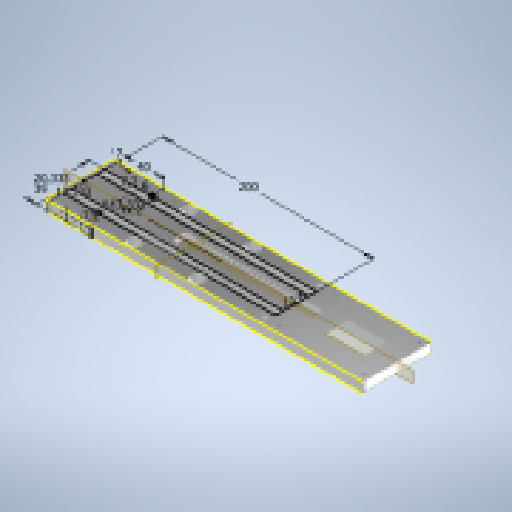
# Autodesk Inventor part: SchlittenS
Saved by Autodesk Inventor 2025 (Build 290162010, 162A)
## iProperties
Created: 2024-11-19
Part Number: SchlittenS
Material: Aluminium 6061(1)
Document SubType Name: Modeling
Designer: Admin
Density: 2.7 g/cm^3
Appearance: Aluminium - flach(1)
Author: Admin
Autodesk Inventor part; units mm, degrees
ref_plane "YZ Plane" through (0, 0, 0) normal (1, 0, 0) x (0, 1, 0)
ref_plane "XZ Plane" through (0, 0, 0) normal (0, 1, 0) x (-1, 0, 0)
ref_plane "XY Plane" through (0, 0, 0) normal (0, 0, 1) x (1, 0, 0)
sketch "Skizze1" plane through (0, 0, 0) normal (0, 0, 1) x (1, 0, 0)
  line L0 (300, 65) -> (0, 65)
  line L1 (0, 65) -> (0, 0)
  line L2 (0, 0) -> (300, 0)
  line L3 (300, 0) -> (300, 65)
  line L4 (144, -16) -> (70, -16)
  line L5 (70, -16) -> (70, 81)
  line L6 (70, 81) -> (144, 81)
  line L7 (144, 81) -> (144, -16)
  dimension "d0" = 300
  dimension "d1" = 65
  dimension "d220" = 74
  dimension "d221" = 16
  dimension "d222" = 16
  dimension "d223" = 70
  constraints: 16 end point, 4 parallel, 2 perpendicular, 1 horizontal, 1 vertical, 1 other
  measures "d0" distance of L2.end L1.end
  measures "d1" distance of L1.end L0.end
  measures "d220" distance of L5.end L6.end
  measures "d221" distance between parallel lines of L2 L4
  measures "d222" distance between parallel lines of L0 L6
  measures "d223" distance between parallel lines of L1 L5
extrude "main" add sketch "Skizze1" along normal blind 10 contours L3 L2 L7 L0 | L7 L2 L5 L0 | L5 L2 L1 L0
sketch "Skizze8" plane through (0, 0, 10) normal (0, 0, 1) x (1, 0, 0)
  line L0 (300, 65) -> (0, 65) projected
  line L1 (0, 65) -> (0, 0) projected
  line L2 (0, 0) -> (300, 0) projected
  line L3 (300, 0) -> (300, 65) projected
  line L4 (77, 6.5) -> (137, 58.5) construction
  line L5 (137, 58.5) -> (137, 6.5) construction
  line L6 (137, 6.5) -> (77, 58.5) construction
  line L7 (77, 58.5) -> (77, 6.5) construction
  line L8 (77, 58.5) -> (137, 58.5) construction
  line L9 (77, 6.5) -> (137, 6.5) construction
  line L10 (77, 6.5) -> (77, 0) construction
  line L11 (77, 58.5) -> (77, 65) construction
  dimension "d30" = 60
  dimension "d88" = 6.5
  dimension "d89" = 77
  constraints: 16 end point, 4 equal length, 3 point on line, 2 parallel, 1 perpendicular
  measures "d30" distance of L5.end L4.start
  measures "d88" distance from line of L2 L4.start
  measures "d89" distance from line of L1 L4.start
hole "BohrungLin" at (77, 6.5, 10) at (137, 6.5, 10) at (137, 58.5, 10) at (77, 58.5, 10) direction (0, 0, -1) diameter 6 end through all countersink diameter 13 countersink angle 90
sketch "Skizze2" plane through (0, 65, 0) normal (0, 1, 0) x (1, 0, 0)
  line L0 (300, 0) -> (0, 0) projected
  line L1 (0, 0) -> (0, -10) projected
  line L2 (7, -7.2) -> (47, -7.2) construction
  point P0 (0, 0)
  dimension "d95" = 7.2
  dimension "d97" = 7
  dimension "d98" = 40
  constraints: 2 end point, 1 coincident, 1 horizontal
  measures "d95" distance from line of L0 L2.start
  measures "d97" distance from line of L1 L2.start
  measures "d98" distance of L2.start L2.end
hole "SeildurchgangR" at (7, 65, 7.2) at (47, 65, 7.2) direction (0, -1, 0) diameter 4 depth 15 tip angle 118
sketch "Skizze4" plane through (0, 0, 0) normal (0, -1, 0) x (1, 0, 0)
  line L0 (33.6667, 7.2) -> (33.6667, 0) construction
  line L1 (20.3333, 7.2) -> (20.3333, 0) construction
  line L2 (0, 0) -> (0, 10) projected
  line L3 (0, 0) -> (300, 0) projected
  dimension "d117" = 7.2
  dimension "d118" = 20.3333
  dimension "d120" = 13.3333
  constraints: 4 end point, 2 coincident, 2 point on line, 1 parallel, 1 perpendicular, 1 vertical
  measures "d117" distance of L0.start L0.end
  measures "d118" distance from line of L2 L1.start
  measures "d120" distance between parallel lines of L0 L1
hole "SeildurchgangL" at (20.3333, 0, 7.2) at (33.6667, 0, 7.2) direction (0, 1, 0) diameter 4 depth 15 tip angle 118
sketch "Skizze10" plane through (0, 0, 10) normal (0, 0, 1) x (1, 0, 0)
  line L0 (204, 13) -> (4, 13)
  line L1 (4, 13) -> (4, 52)
  line L2 (4, 52) -> (204, 52)
  line L3 (204, 52) -> (204, 13)
  circle A0 centre (35.6667, 13) radius 3
  circle A1 centre (49, 52) radius 3
  line L4 (4, 52) -> (4, 65) construction
  line L5 (4, 13) -> (4, 0) construction
  line L6 (35.6667, 13) -> (35.6667, 52) construction
  line L7 (300, 65) -> (0, 65) projected
  line L8 (0, 65) -> (0, 0) projected
  line L9 (0, 0) -> (300, 0) projected
  line L10 (77, 65) -> (0, 65) projected
  line L11 (0, 0) -> (77, 0) projected
  line L12 (45, 65) -> (49, 65) projected
  line L13 (47, 65) -> (47, 52) construction
  line L14 (204, 20.5) -> (4, 20.5)
  line L15 (4, 20.5) -> (4, 44.5)
  line L16 (4, 44.5) -> (204, 44.5)
  line L17 (204, 44.5) -> (204, 20.5)
  line L18 (204, 32.5) -> (204, 44.5) construction
  line L19 (204, 32.5) -> (204, 20.5) construction
  point P0 (4, 32.5)
  point P1 (-264.0828, -97.6171)
  point P2 (-272.0828, -97.6171)
  point P3 (-285.4161, -110.6171)
  point P4 (-277.4161, -110.6171)
  point P5 (204, 44.5)
  point P6 (4, 20.5)
  dimension "d45" = 39
  dimension "d70" = 6
  dimension "d73" = 6
  dimension "d91" = 200
  dimension "d92" = 13.3333
  dimension "d99" = 4
  dimension "d100" = 2
  dimension "d161" = 12
  constraints: 31 end point, 11 point on line, 6 perpendicular, 4 midpoint, 4 parallel, 2 centre point, 2 collinear, 2 horizontal, 1 vertical
  measures "d45" distance of L1.end L0.end
  measures "d70" diameter of A0
  measures "d73" diameter of A1
  measures "d91" distance of point (4, 32.5) L18.start
  measures "d92" distance from line of A1.centre L6
  measures "d99" distance from line of L8 point (4, 32.5)
  measures "d100" distance of L13.end A1.centre
  measures "d161" distance from line of L16 point (204, 32.5)
extrude "SeilUmlenkAussparung" cut sketch "Skizze10" against normal blind 5 contours L0 A0 L1 L14 L3 | A0 L0 | L0 A0 | L16 L1 L2 A1 L3 | A1 L2 | L2 A1
sketch "Skizze11" plane through (0, 0, 5) normal (0, 0, 1) x (1, 0, 0)
  arc A0 (52, 52) -> (46, 52) centre (49, 52) ccw construction
  arc A1 (32.6667, 13) -> (38.6667, 13) centre (35.6667, 13) ccw construction
  line L0 (35.6667, 14) -> (35.6667, 16) construction
  line L1 (35.6667, 16) -> (35.6667, 25.6667) construction
  line L2 (35.6667, 25.6667) -> (35.6667, 27.6667) construction
  line L3 (35.6667, 27.6667) -> (35.6667, 37.3333) construction
  line L4 (35.6667, 37.3333) -> (35.6667, 39.3333) construction
  line L5 (35.6667, 39.3333) -> (35.6667, 49) construction
  line L6 (35.6667, 49) -> (35.6667, 51) construction
  line L7 (49, 52) -> (35.6667, 52) construction
  line L8 (35.6667, 14) -> (35.6667, 13) construction
  line L9 (35.6667, 51) -> (35.6667, 52) construction
  line L10 (9, 49) -> (35.6667, 49) construction
  line L11 (22.3333, 16) -> (35.6667, 16) construction
  point P0 (49, 52)
  point P1 (35.6667, 13)
  dimension "d103" = 9.6667
  dimension "d104" = 9.6667
  dimension "d107" = 2
  dimension "d108" = 2
  dimension "d109" = 2
  dimension "d110" = 1
  dimension "d111" = 1
  dimension "d112" = 2
  dimension "d114" = 13.3333
  dimension "d115" = 13.3333
  dimension "d116" = 13.3333
  constraints: 24 end point, 6 point on line, 5 collinear, 3 horizontal, 3 vertical, 2 coincident
  measures "d103" distance of L2.end L3.end
  measures "d104" distance of L4.end L5.end
  measures "d107" distance of L1.end L2.end
  measures "d108" distance of L3.end L4.end
  measures "d109" distance of L6.end L5.end
  measures "d110" distance of L0.start L8.end
  measures "d111" distance of L6.end L7.end
  measures "d112" distance of L0.start L0.end
  measures "d114" distance of L7.start L7.end
  measures "d115" distance from line of L6 L11.start
  measures "d116" horizontal distance of L11.start L10.start
hole "stifte" at (9, 49, 5) at (49, 52, 5) at (35.6667, 13, 5) at (22.3333, 16, 5) direction (0, 0, -1) diameter 2 depth 2 tip angle 118
sketch "Skizze12" plane through (0, 0, 0) normal (0, 0, -1) x (-1, 0, 0)
  circle A0 centre (-77, 58.5) radius 3 projected
  circle A1 centre (-137, 58.5) radius 3 projected
  circle A2 centre (-137, 6.5) radius 3 projected
  circle A3 centre (-77, 6.5) radius 3 projected
  line L0 (0, 0) -> (-300, 0) projected
  line L1 (0, 65) -> (0, 0) projected
  line L2 (-300, 65) -> (0, 65) projected
  line L3 (-300, 0) -> (-300, 65) projected
  line L4 (-137, 6.5) -> (-77, 6.5) construction
  line L5 (-107, 6.5) -> (-107, 58.5) construction
  line L6 (-117.5, 4) -> (-96.5, 4)
  line L7 (-96.5, 4) -> (-96.5, 9)
  line L8 (-96.5, 9) -> (-117.5, 9)
  line L9 (-117.5, 9) -> (-117.5, 4)
  line L10 (-117.5, 9) -> (-107, 9) construction
  line L11 (-107, 9) -> (-96.5, 9) construction
  line L12 (-107, 32.5) -> (-127, 32.5) construction
  line L13 (-137, 58.5) -> (-77, 58.5) construction
  line L14 (-117.5, 61) -> (-96.5, 61)
  line L15 (-96.5, 61) -> (-96.5, 56)
  line L16 (-96.5, 56) -> (-117.5, 56)
  line L17 (-117.5, 56) -> (-117.5, 61)
  dimension "d125" = 21
  dimension "d126" = 5
  dimension "d127" = 4
  dimension "d128" = 20
  constraints: 28 end point, 5 horizontal, 4 symmetric about line, 3 midpoint, 2 parallel, 1 collinear, 1 perpendicular, 1 point on line, 1 vertical
  measures "d125" distance of L8.end L7.end
  measures "d126" distance of L7.end L6.end
  measures "d127" distance between parallel lines of L0 L6
  measures "d128" distance of L12.start L12.end
extrude "Extrusion7" cut sketch "Skizze12" against normal blind 3.5 contours L9 L8 L7 L6 | L14 L15 L16 L17
fillet "Rundung1" radius 2.5 4 edges at (107, 9, 3.5) (107, 61, 3.5) (107, 4, 3.5) (107, 56, 3.5)
chamfer "Fasen1" distance 1 angle 45 4 edges at (107, 61, 0) (107, 56, 0) (107, 4, 0) (107, 9, 0)
sketch "Skizze13" plane through (117.5, 3, 0) normal (-1, 0, 0) x (0, 0, 1)
  arc A0 (1, 1) -> (1, 6) centre (1, 3.5) ccw projected
  arc A1 (1, 53) -> (1, 58) centre (1, 55.5) ccw projected
  circle A2 centre (1, 3.5) radius 1
  line L0 (1, 2.5) -> (0, 2.5)
  line L1 (0, 2.5) -> (0, 4.5)
  line L2 (0, 4.5) -> (1, 4.5)
  line L3 (1, 4.5) -> (1, 2.5)
  circle A3 centre (1, 55.5) radius 1
  line L4 (0, 52) -> (0, 59) projected
  line L5 (1, 54.5) -> (0, 54.5)
  line L6 (0, 54.5) -> (0, 56.5)
  line L7 (0, 56.5) -> (1, 56.5)
  line L8 (1, 56.5) -> (1, 54.5)
  point P0 (0, -3)
  point P1 (0, 3.5)
  dimension "d135" = 2
  dimension "d136" = 1
  dimension "d137" = 2
  constraints: 16 end point, 5 horizontal, 4 coincident, 4 parallel, 2 perpendicular, 1 point on line, 1 vertical, 6 other
  measures "d136" distance of L1.end L2.end
  measures "d137" distance of L0.end L1.end
extrude "Extrusion8" cut sketch "Skizze13" against normal blind 5
ref_plane "Arbeitsebene1" through (107, 6.5, 1) normal (-1, 0, 0) x (0, 0, 1)
mirror "Spiegeln1" about plane through (107, 6.5, 1) normal (-1, 0, 0) of "Extrusion8"
sketch "Skizze14" plane through (0, 0, 0) normal (0, 0, -1) x (-1, 0, 0)
  line L0 (-77, 0) -> (-137, 0) construction
  line L1 (-107, 0) -> (-107, 29) construction
  line L2 (-107, 29) -> (-102.75, 29) construction
  line L3 (-102.75, 29) -> (-102.75, 27.25) construction
  line L4 (-107, 29) -> (-111.25, 29) construction
  line L5 (-111.25, 29) -> (-111.25, 27.25) construction
  line L6 (-102.75, 23.75) -> (-102.75, 27.25) construction
  line L7 (-111.25, 23.75) -> (-111.25, 27.25) construction
  point P0 (0, 0)
  dimension "d140" = 29
  dimension "d141" = 4.25
  dimension "d142" = 1.75
  dimension "d143" = 3.5
  constraints: 14 end point, 3 equal length, 3 perpendicular, 3 vertical, 2 coincident, 1 horizontal, 1 midpoint
  measures "d140" distance of L1.start L1.end
  measures "d141" distance of L1.end L2.end
  measures "d142" distance of L2.end L3.end
  measures "d143" distance of L6.start L6.end
hole "Bohrung6" at (102.75, 23.75, 0) at (102.75, 27.25, 0) at (111.25, 23.75, 0) at (111.25, 27.25, 0) direction (0, 0, 1) diameter 1.567 depth 6.3 tip angle 118
ref_plane "Arbeitsebene2" through (0, 32.5, 0) normal (0, -1, 0) x (1, 0, 0)
mirror "Spiegeln2" about plane through (0, 32.5, 0) normal (0, -1, 0) of "Bohrung6"
sketch "Skizze15" plane through (0, 0, 0) normal (0, 0, -1) x (-1, 0, 0)
  line L0 (-137, 6.5) -> (-137, 58.5) construction
  line L1 (60, 32.5) -> (-360, 32.5) construction
  line L2 (-145.5, 36.75) -> (-152, 36.75) construction
  line L3 (-145.5, 28.25) -> (-152, 28.25) construction
  circle A0 centre (-137, 58.5) radius 3 projected
  circle A1 centre (-137, 6.5) radius 3 projected
  line L4 (-172, 48.1296) -> (-172, 10.7181) construction
  line L5 (-225.5, 29.25) -> (-225.5, 32.5) construction
  line L6 (-225.5, 32.5) -> (-225.5, 35.75) construction
  line L7 (-107, 78) -> (-107, -13) construction
  point P0 (0, 0)
  point P1 (-192, 36.75)
  point P2 (-198.5, 36.75)
  point P3 (-198.5, 28.25)
  point P4 (-192, 28.25)
  point P5 (-62, 36.75)
  point P6 (-68.5, 36.75)
  point P7 (-68.5, 28.25)
  point P8 (-62, 28.25)
  dimension "d151" = 15
  dimension "d152" = 6.5
  dimension "d153" = 4.25
  dimension "d215" = 20
  dimension "d217" = 6.5
  dimension "d219" = 27
  constraints: 12 end point, 10 symmetric about line, 2 coincident, 2 collinear, 2 parallel, 1 perpendicular, 1 point on line
  measures "d151" distance from line of L0 L2.end
  measures "d152" distance of L2.start L2.end
  measures "d153" distance from line of L1 L2.end
  measures "d215" distance from line of L3.end L4
  measures "d217" distance of L6.end L5.start
  measures "d219" distance from line of point (-198.5, 28.25) L5
hole "Bohrung7" at (152, 36.75, 0) at (145.5, 36.75, 0) at (145.5, 28.25, 0) at (152, 28.25, 0) at (192, 36.75, 0) at (192, 28.25, 0) at (198.5, 28.25, 0) at (198.5, 36.75, 0) at (225.5, 35.75, 0) at (225.5, 29.25, 0) at (68.5, 36.75, 0) at (62, 36.75, 0) at (62, 28.25, 0) at (68.5, 28.25, 0) direction (0, 0, 1) diameter 1.567 depth 6.3 tip angle 118
fillet "Rundung2" radius 3 8 edges at (4, 13, 7.5) (4, 44.5, 7.5) (4, 20.5, 7.5) (4, 52, 7.5) (204, 20.5, 7.5) (204, 52, 7.5) (204, 13, 7.5) (204, 44.5, 7.5)
sketch "Skizze16" plane through (0, 0, 10) normal (0, 0, 1) x (1, 0, 0)
  line L0 (93.5, 25.5) -> (224, 25.5)
  line L1 (224, 25.5) -> (224, 39.5)
  line L2 (224, 39.5) -> (93.5, 39.5)
  line L3 (93.5, 39.5) -> (93.5, 25.5)
  line L4 (93.5, 25.5) -> (93.5, 20.5) construction
  line L5 (7, 20.5) -> (201, 20.5) construction
  line L6 (93.5, 39.5) -> (93.5, 44.5) construction
  line L7 (201, 44.5) -> (7, 44.5) construction
  arc A0 (77, 52) -> (77, 65) centre (77, 58.5) ccw construction
  line L8 (204, 49) -> (204, 47.5) construction
  point P0 (0, 0)
  point P1 (83.5, 58.5)
  point P2 (204, 48.25)
  dimension "d163" = 5
  dimension "d164" = 10
  dimension "d165" = 20
  constraints: 12 end point, 2 parallel, 2 perpendicular, 2 point on line, 1 collinear, 1 horizontal, 1 midpoint, 1 point on circle, 1 vertical
  measures "d163" distance of L0.start L4.end
  measures "d164" distance from line of point (83.5, 58.5) L3
  measures "d165" distance from line of point (204, 48.25) L1
extrude "Extrusion9" cut sketch "Skizze16" against normal blind 5
fillet "Rundung3" radius 3 4 edges at (93.5, 25.5, 7.5) (93.5, 39.5, 7.5) (224, 25.5, 7.5) (224, 39.5, 7.5)
sketch "Skizze17" plane through (0, 0, 10) normal (0, 0, 1) x (1, 0, 0)
  line L0 (108.5, 20.5) -> (111, 20.5)
  line L1 (111, 20.5) -> (111, 25.5)
  line L2 (111, 25.5) -> (108.5, 25.5)
  line L3 (108.5, 25.5) -> (108.5, 20.5)
  line L4 (93.5, 28.5) -> (93.5, 36.5) projected
  line L5 (96.5, 39.5) -> (221, 39.5) projected
  line L6 (204, 20.5) -> (4, 20.5) projected
  line L7 (4, 44.5) -> (204, 44.5) projected
  line L8 (108.5, 20.5) -> (111, 20.5)
  line L9 (116, 25.5) -> (113.5, 25.5)
  line L10 (113.5, 25.5) -> (113.5, 20.5)
  line L11 (113.5, 20.5) -> (116, 20.5)
  line L12 (116, 20.5) -> (116, 25.5)
  line L13 (121, 25.5) -> (118.5, 25.5)
  line L14 (118.5, 25.5) -> (118.5, 20.5)
  line L15 (118.5, 20.5) -> (121, 20.5)
  line L16 (121, 20.5) -> (121, 25.5)
  line L17 (126, 25.5) -> (123.5, 25.5)
  line L18 (123.5, 25.5) -> (123.5, 20.5)
  line L19 (123.5, 20.5) -> (126, 20.5)
  line L20 (126, 20.5) -> (126, 25.5)
  line L21 (131, 25.5) -> (128.5, 25.5)
  line L22 (128.5, 25.5) -> (128.5, 20.5)
  line L23 (128.5, 20.5) -> (131, 20.5)
  line L24 (131, 20.5) -> (131, 25.5)
  line L25 (136, 25.5) -> (133.5, 25.5)
  line L26 (133.5, 25.5) -> (133.5, 20.5)
  line L27 (133.5, 20.5) -> (136, 20.5)
  line L28 (136, 20.5) -> (136, 25.5)
  line L29 (141, 25.5) -> (138.5, 25.5)
  line L30 (138.5, 25.5) -> (138.5, 20.5)
  line L31 (138.5, 20.5) -> (141, 20.5)
  line L32 (141, 20.5) -> (141, 25.5)
  line L33 (146, 25.5) -> (143.5, 25.5)
  line L34 (143.5, 25.5) -> (143.5, 20.5)
  line L35 (143.5, 20.5) -> (146, 20.5)
  line L36 (146, 20.5) -> (146, 25.5)
  line L37 (151, 25.5) -> (148.5, 25.5)
  line L38 (148.5, 25.5) -> (148.5, 20.5)
  line L39 (148.5, 20.5) -> (151, 20.5)
  line L40 (151, 20.5) -> (151, 25.5)
  line L41 (156, 25.5) -> (153.5, 25.5)
  line L42 (153.5, 25.5) -> (153.5, 20.5)
  line L43 (153.5, 20.5) -> (156, 20.5)
  line L44 (156, 20.5) -> (156, 25.5)
  line L45 (161, 25.5) -> (158.5, 25.5)
  line L46 (158.5, 25.5) -> (158.5, 20.5)
  line L47 (158.5, 20.5) -> (161, 20.5)
  line L48 (161, 20.5) -> (161, 25.5)
  line L49 (166, 25.5) -> (163.5, 25.5)
  line L50 (163.5, 25.5) -> (163.5, 20.5)
  line L51 (163.5, 20.5) -> (166, 20.5)
  line L52 (166, 20.5) -> (166, 25.5)
  line L53 (171, 25.5) -> (168.5, 25.5)
  line L54 (168.5, 25.5) -> (168.5, 20.5)
  line L55 (168.5, 20.5) -> (171, 20.5)
  line L56 (171, 20.5) -> (171, 25.5)
  line L57 (176, 25.5) -> (173.5, 25.5)
  line L58 (173.5, 25.5) -> (173.5, 20.5)
  line L59 (173.5, 20.5) -> (176, 20.5)
  line L60 (176, 20.5) -> (176, 25.5)
  line L61 (181, 25.5) -> (178.5, 25.5)
  line L62 (178.5, 25.5) -> (178.5, 20.5)
  line L63 (178.5, 20.5) -> (181, 20.5)
  line L64 (181, 20.5) -> (181, 25.5)
  line L65 (186, 25.5) -> (183.5, 25.5)
  line L66 (183.5, 25.5) -> (183.5, 20.5)
  line L67 (183.5, 20.5) -> (186, 20.5)
  line L68 (186, 20.5) -> (186, 25.5)
  line L69 (191, 25.5) -> (188.5, 25.5)
  line L70 (188.5, 25.5) -> (188.5, 20.5)
  line L71 (188.5, 20.5) -> (191, 20.5)
  line L72 (191, 20.5) -> (191, 25.5)
  line L73 (196, 25.5) -> (193.5, 25.5)
  line L74 (193.5, 25.5) -> (193.5, 20.5)
  line L75 (193.5, 20.5) -> (196, 20.5)
  line L76 (196, 20.5) -> (196, 25.5)
  line L77 (111, 44.5) -> (108.5, 44.5)
  line L78 (108.5, 44.5) -> (108.5, 39.5)
  line L79 (108.5, 39.5) -> (111, 39.5)
  line L80 (111, 39.5) -> (111, 44.5)
  line L81 (116, 44.5) -> (113.5, 44.5)
  line L82 (113.5, 44.5) -> (113.5, 39.5)
  line L83 (113.5, 39.5) -> (116, 39.5)
  line L84 (116, 39.5) -> (116, 44.5)
  line L85 (121, 44.5) -> (118.5, 44.5)
  line L86 (118.5, 44.5) -> (118.5, 39.5)
  line L87 (118.5, 39.5) -> (121, 39.5)
  line L88 (121, 39.5) -> (121, 44.5)
  line L89 (126, 44.5) -> (123.5, 44.5)
  line L90 (123.5, 44.5) -> (123.5, 39.5)
  line L91 (123.5, 39.5) -> (126, 39.5)
  line L92 (126, 39.5) -> (126, 44.5)
  line L93 (131, 44.5) -> (128.5, 44.5)
  line L94 (128.5, 44.5) -> (128.5, 39.5)
  line L95 (128.5, 39.5) -> (131, 39.5)
  line L96 (131, 39.5) -> (131, 44.5)
  line L97 (136, 44.5) -> (133.5, 44.5)
  line L98 (133.5, 44.5) -> (133.5, 39.5)
  line L99 (133.5, 39.5) -> (136, 39.5)
  line L100 (136, 39.5) -> (136, 44.5)
  line L101 (141, 44.5) -> (138.5, 44.5)
  line L102 (138.5, 44.5) -> (138.5, 39.5)
  line L103 (138.5, 39.5) -> (141, 39.5)
  line L104 (141, 39.5) -> (141, 44.5)
  line L105 (146, 44.5) -> (143.5, 44.5)
  line L106 (143.5, 44.5) -> (143.5, 39.5)
  line L107 (143.5, 39.5) -> (146, 39.5)
  line L108 (146, 39.5) -> (146, 44.5)
  line L109 (151, 44.5) -> (148.5, 44.5)
  line L110 (148.5, 44.5) -> (148.5, 39.5)
  line L111 (148.5, 39.5) -> (151, 39.5)
  line L112 (151, 39.5) -> (151, 44.5)
  line L113 (156, 44.5) -> (153.5, 44.5)
  line L114 (153.5, 44.5) -> (153.5, 39.5)
  line L115 (153.5, 39.5) -> (156, 39.5)
  line L116 (156, 39.5) -> (156, 44.5)
  line L117 (161, 44.5) -> (158.5, 44.5)
  line L118 (158.5, 44.5) -> (158.5, 39.5)
  line L119 (158.5, 39.5) -> (161, 39.5)
  line L120 (161, 39.5) -> (161, 44.5)
  line L121 (166, 44.5) -> (163.5, 44.5)
  line L122 (163.5, 44.5) -> (163.5, 39.5)
  line L123 (163.5, 39.5) -> (166, 39.5)
  line L124 (166, 39.5) -> (166, 44.5)
  line L125 (171, 44.5) -> (168.5, 44.5)
  line L126 (168.5, 44.5) -> (168.5, 39.5)
  line L127 (168.5, 39.5) -> (171, 39.5)
  line L128 (171, 39.5) -> (171, 44.5)
  line L129 (176, 44.5) -> (173.5, 44.5)
  line L130 (173.5, 44.5) -> (173.5, 39.5)
  line L131 (173.5, 39.5) -> (176, 39.5)
  line L132 (176, 39.5) -> (176, 44.5)
  line L133 (181, 44.5) -> (178.5, 44.5)
  line L134 (178.5, 44.5) -> (178.5, 39.5)
  line L135 (178.5, 39.5) -> (181, 39.5)
  line L136 (181, 39.5) -> (181, 44.5)
  line L137 (186, 44.5) -> (183.5, 44.5)
  line L138 (183.5, 44.5) -> (183.5, 39.5)
  line L139 (183.5, 39.5) -> (186, 39.5)
  line L140 (186, 39.5) -> (186, 44.5)
  line L141 (191, 44.5) -> (188.5, 44.5)
  line L142 (188.5, 44.5) -> (188.5, 39.5)
  line L143 (188.5, 39.5) -> (191, 39.5)
  line L144 (191, 39.5) -> (191, 44.5)
  line L145 (196, 44.5) -> (193.5, 44.5)
  line L146 (193.5, 44.5) -> (193.5, 39.5)
  line L147 (193.5, 39.5) -> (196, 39.5)
  line L148 (196, 39.5) -> (196, 44.5)
  line L149 (221, 25.5) -> (96.5, 25.5) projected
  point P0 (0, 0)
  point P1 (193.5, 20.5)
  point P2 (196, 20.5)
  point P3 (188.5, 20.5)
  point P4 (191, 20.5)
  point P5 (183.5, 20.5)
  point P6 (186, 20.5)
  point P7 (178.5, 20.5)
  point P8 (181, 20.5)
  point P9 (173.5, 20.5)
  point P10 (168.5, 20.5)
  point P11 (163.5, 20.5)
  point P12 (158.5, 20.5)
  point P13 (153.5, 20.5)
  point P14 (148.5, 20.5)
  point P15 (151, 20.5)
  point P16 (143.5, 20.5)
  point P17 (146, 20.5)
  point P18 (141, 20.5)
  point P19 (136, 20.5)
  point P20 (131, 20.5)
  point P21 (126, 20.5)
  point P22 (166, 39.5)
  point P23 (166, 44.5)
  point P24 (163.5, 44.5)
  point P25 (163.5, 39.5)
  point P26 (171, 39.5)
  point P27 (171, 44.5)
  point P28 (168.5, 44.5)
  point P29 (168.5, 39.5)
  point P30 (176, 39.5)
  point P31 (176, 44.5)
  point P32 (173.5, 44.5)
  point P33 (173.5, 39.5)
  point P34 (181, 39.5)
  point P35 (181, 44.5)
  point P36 (178.5, 44.5)
  point P37 (178.5, 39.5)
  point P38 (186, 39.5)
  point P39 (186, 44.5)
  point P40 (183.5, 44.5)
  point P41 (183.5, 39.5)
  point P42 (191, 39.5)
  point P43 (191, 44.5)
  point P44 (188.5, 44.5)
  point P45 (196, 44.5)
  point P46 (193.5, 44.5)
  point P47 (161, 39.5)
  point P48 (161, 44.5)
  point P49 (158.5, 44.5)
  point P50 (158.5, 39.5)
  point P51 (156, 39.5)
  point P52 (156, 44.5)
  point P53 (153.5, 44.5)
  point P54 (153.5, 39.5)
  point P55 (151, 39.5)
  point P56 (151, 44.5)
  point P57 (148.5, 44.5)
  point P58 (148.5, 39.5)
  point P59 (146, 39.5)
  point P60 (146, 44.5)
  point P61 (143.5, 44.5)
  point P62 (143.5, 39.5)
  point P63 (141, 39.5)
  point P64 (141, 44.5)
  point P65 (138.5, 44.5)
  point P66 (138.5, 39.5)
  point P67 (136, 39.5)
  point P68 (136, 44.5)
  point P69 (133.5, 44.5)
  point P70 (133.5, 39.5)
  point P71 (131, 39.5)
  point P72 (131, 44.5)
  point P73 (128.5, 44.5)
  point P74 (128.5, 39.5)
  point P75 (126, 39.5)
  point P76 (126, 44.5)
  point P77 (123.5, 44.5)
  point P78 (123.5, 39.5)
  point P79 (121, 39.5)
  point P80 (121, 44.5)
  point P81 (118.5, 44.5)
  point P82 (118.5, 39.5)
  point P83 (116, 39.5)
  point P84 (116, 44.5)
  point P85 (113.5, 44.5)
  point P86 (113.5, 39.5)
  point P87 (111, 39.5)
  point P88 (111, 44.5)
  point P89 (108.5, 44.5)
  point P90 (108.5, 39.5)
  point P91 (121, 20.5)
  point P92 (113.5, 20.5)
  point P93 (116, 20.5)
  dimension "d169" = 2.5
  dimension "d170" = 15
  dimension "d181" = 5
  dimension "d184" = 19
  constraints: 290 end point, 68 horizontal alignment, 36 parallel, 35 collinear, 3 horizontal, 1 perpendicular, 1 vertical, 147 other
  measures "d169" distance of L2.end L1.end
  measures "d170" distance between parallel lines of L4 L3
  measures "d181" distance of L1.end L9.start
  measures "d184" distance of L1.end L77.start
sketch "Skizze18" plane through (98.9767, 25.5, 5) normal (0, 1, 0) x (1, 0, 0)
  line L0 (12.0233, -5) -> (10.0233, -1.5359)
  line L1 (12.0233, -5) -> (16.0233, -5) construction
  point P0 (-98.9767, 5)
  dimension "d187" = 4
  dimension "d188" = 120
  constraints: 4 end point, 1 equal length, 1 horizontal
  measures "d187" distance of L0.start L0.end
  measures "d188" angle of L1 L0
sweep "Sweeping1" cut profiles "Skizze17" path "Skizze18" contours L3 L2 L1 L0 | L10 L9 L12 L6 | L14 L13 L16 L6 | L18 L17 L20 L6 | L22 L21 L24 L6 | L26 L25 L28 L6 | L30 L29 L32 L6 | L34 L33 L36 L6 | L38 L37 L40 L6 | L42 L41 L44 L6 | L46 L45 L48 L6 | L50 L49 L52 L6 | L54 L53 L56 L6 | L58 L57 L60 L6 | L62 L61 L64 L6 | L66 L65 L68 L6 | L70 L69 L72 L6 | L74 L73 L76 L6 | L78 L7 L80 L5 | L82 L7 L84 L5 | L86 L7 L88 L5 | L90 L7 L92 L5 | L94 L7 L96 L5 | L98 L7 L100 L5 | L102 L7 L104 L5 | L106 L7 L108 L5 | L110 L7 L112 L5 | L114 L7 L116 L5 | L118 L7 L120 L5 | L122 L7 L124 L5 | L126 L7 L128 L5 | L130 L7 L132 L5 | L134 L7 L136 L5 | L138 L7 L140 L5 | L142 L7 L144 L5 | L146 L7 L148 L5
fillet "Rundung4" radius 2 8 edges at (300, 65, 5) (300, 32.5, 0) (150, 65, 0) (0, 65, 5) (0, 32.5, 0) (0, 0, 5) (150, 0, 0) (300, 0, 5)
sketch "Skizze19" plane through (0, 0, 10) normal (0, 0, 1) x (1, 0, 0)
  circle A0 centre (294, 59) radius 1.6 projected
  circle A1 centre (294, 6) radius 1.6 projected
  circle A2 centre (214, 59) radius 1.6 projected
  circle A3 centre (214, 6) radius 1.6 projected
  point P0 (0, 0)
hole "Bohrung8" at (294, 6, 10) at (294, 59, 10) at (214, 59, 10) at (214, 6, 10) direction (0, 0, -1) diameter 2.459 depth 7.8 tip angle 118
sketch "Skizze20" plane through (0, 0, 10) normal (0, 0, 1) x (1, 0, 0)
  circle A0 centre (62, 59) radius 1.6 projected
  circle A1 centre (6, 32.5) radius 1.6 projected
  circle A2 centre (62, 6) radius 1.6 projected
  circle A3 centre (90.5, 25) radius 1.6 projected
  circle A4 centre (90.5, 40) radius 1.6 projected
  point P0 (0, 0)
hole "Bohrung9" at (6, 32.5, 10) at (62, 59, 10) at (90.5, 40, 10) at (90.5, 25, 10) at (62, 6, 10) direction (0, 0, -1) diameter 2.459 depth 7.8 tip angle 118
sketch "Skizze22" plane through (0, 0, 10) normal (0, 0, 1) x (1, 0, 0)
  line L0 (278.64, 43.5) -> (243, 43.5) projected
  line L1 (243, 21.5) -> (243, 43.5) projected
  line L2 (278.64, 21.5) -> (243, 21.5) projected
  line L3 (278.64, 21.5) -> (278.64, 43.5) projected
  line L4 (278.64, 43.5) -> (243, 43.5) projected
  point P0 (0, 0)
sketch "Skizze23" plane through (0, 0, 0) normal (0, 0, -1) x (-1, 0, 0)
  line L0 (-282, 48.5) -> (-246, 16.5) construction
  line L1 (-246, 48.5) -> (-282, 16.5) construction
  line L2 (-249, 32.5) -> (-248, 32.5) construction
  line L3 (-249, 42.5) -> (-275.82, 42.5) construction
  line L4 (-275.82, 22.5) -> (-249, 22.5) construction
  line L5 (-281.28, 22.5) -> (-234, 22.5) construction
  line L6 (-234, 22.5) -> (-234, 42.5) construction
  line L7 (-234, 42.5) -> (-281.28, 42.5) construction
  line L8 (-281.28, 42.5) -> (-281.28, 22.5) construction
  line L9 (-282.28, 21.5) -> (-233, 21.5)
  line L10 (-233, 21.5) -> (-233, 43.5)
  line L11 (-233, 43.5) -> (-282.28, 43.5)
  line L12 (-282.28, 43.5) -> (-282.28, 21.5)
  line L13 (-281.28, 32.5) -> (-282.28, 32.5) construction
  line L14 (-234, 32.5) -> (-233, 32.5) construction
  line L15 (-257.64, 42.5) -> (-257.64, 43.5) construction
  line L16 (-257.64, 22.5) -> (-257.64, 21.5) construction
  point P0 (0, 0)
  point P1 (-264, 32.5)
  dimension "d206" = 17.28
  dimension "d207" = 30
  constraints: 24 end point, 8 midpoint, 4 equal length, 4 parallel, 4 perpendicular, 2 collinear, 2 horizontal, 1 point on line
  measures "d206" distance from line of L8 point (-264, 32.5)
  measures "d207" distance of L14.start point (-264, 32.5)
loft "Erhebung1" cut profiles "Skizze22", "Skizze23"
sketch "Skizze24" plane through (0, 0, 10) normal (0, 0, 1) x (1, 0, 0)
  circle A0 centre (200.6132, 58.5) radius 2.65
  line L0 (200.6132, 58.5) -> (200.6132, 65) construction
  line L1 (298, 65) -> (137, 65) construction
  line L2 (200.6132, 58.5) -> (200.6132, 52) construction
  line L3 (137, 52) -> (201, 52) construction
  line L4 (200.6132, 58.5) -> (207.1132, 58.5) construction
  line L5 (207.1132, 42) -> (207.1132, 65) construction
  line L6 (137, 0) -> (298, 0) construction
  line L7 (200.6132, 0) -> (200.6132, 6.5) construction
  line L8 (200.6132, 6.5) -> (200.6132, 13) construction
  line L9 (200.6132, 6.5) -> (207.1132, 6.5) construction
  line L10 (207.1132, 0) -> (207.1132, 23) construction
  line L11 (201, 13) -> (137, 13) construction
  circle A1 centre (200.6132, 6.5) radius 2.65
  line L12 (200.6132, 6.5) -> (197.9632, 6.5) construction
  line L13 (298, 0) -> (2, 0) construction
  line L14 (200.6132, 58.5) -> (197.9632, 58.5) construction
  point P0 (0, 0)
  dimension "d212" = 5.3
  constraints: 16 end point, 8 point on line, 6 equal length, 2 horizontal, 2 horizontal alignment, 2 vertical, 1 coincident, 1 parallel, 1 perpendicular, 4 other
extrude "Extrusion10" cut sketch "Skizze24" against normal blind 3.3
